Autodesk Inventor part; units mm, degrees
note: some values were not read from the file. Chosen so that the rebuilt part matches the saved one: direction of "Hole2".
(part 3 of 3)
  spline S120 degree 3 poles (-3.4442, 27.3191) (-3.5354, 27.4125) (-3.6453, 27.4727) (-3.7727, 27.4993) (-3.9002, 27.526) (-4.0253, 27.5146) (-4.1459, 27.4656) (-4.2665, 27.4166) (-4.3639, 27.3373) (-4.4367, 27.2293) (-4.5094, 27.1213) (-4.546, 27.0018) (-4.5461, 26.8709) knots 0 0 0 0 0.25 0.25 0.25 0.5 0.5 0.5 0.75 0.75 0.75 1 1 1 1
  spline S121 degree 3 poles (-5.388, 28.9585) (-5.3885, 28.9241) (-5.3861, 28.89) (-5.3809, 28.8564) knots 0 0 0 0 1 1 1 1
  line L115 (-4.5538, 28.7429) -> (-4.7042, 28.7429)
  spline S122 degree 3 poles (-5.3809, 28.8564) (-5.3777, 28.8422) (-5.3745, 28.8314) (-5.3727, 28.8257) (-5.3723, 28.8246) (-5.372, 28.8238) (-5.372, 28.8238) (-5.3718, 28.8234) (-5.3717, 28.8232) (-5.3716, 28.823) (-5.3715, 28.823) (-5.3715, 28.8229) (-5.3715, 28.8229) (-5.3715, 28.8229) (-5.3715, 28.8229) (-5.3715, 28.8229) (-5.3715, 28.8229) (-5.3715, 28.8229) (-5.3715, 28.8229) (-5.3715, 28.8229) (-5.3715, 28.823) (-5.3714, 28.823) (-5.3714, 28.823) (-5.3714, 28.8231) (-5.3714, 28.8232) (-5.3715, 28.8244) (-5.3721, 28.8277) (-5.3775, 28.8551) (-5.3859, 28.896) (-5.388, 28.9585) knots 0 0 0 0 0.216458 0.216458 0.250147 0.250147 0.25213 0.25213 0.266562 0.266562 0.270758 0.270758 0.271952 0.271952 0.272738 0.272738 0.27341 0.27341 0.274154 0.274154 0.275352 0.275352 0.277883 0.277883 0.289351 0.289351 0.40678 0.40678 1 1 1 1
  line L116 (-4.7883, 28.3589) -> (-4.4696, 28.3589)
  line L117 (-4.7883, 28.3589) -> (-4.4696, 28.3589)
  spline S123 degree 3 poles (-4.4696, 28.3589) (-4.4353, 28.359) (-4.4013, 28.3621) (-4.3679, 28.3678) knots 0 0 0 0 1 1 1 1
  spline S124 degree 3 poles (-4.3679, 28.3678) (-4.3538, 28.3714) (-4.343, 28.3747) (-4.3374, 28.3767) (-4.3363, 28.3771) (-4.3355, 28.3774) (-4.3355, 28.3774) (-4.3351, 28.3776) (-4.3349, 28.3777) (-4.3347, 28.3778) (-4.3347, 28.3779) (-4.3346, 28.3779) (-4.3346, 28.3779) (-4.3346, 28.3779) (-4.3346, 28.3779) (-4.3346, 28.3779) (-4.3346, 28.3779) (-4.3346, 28.3779) (-4.3346, 28.3779) (-4.3347, 28.3779) (-4.3347, 28.3779) (-4.3347, 28.378) (-4.3347, 28.378) (-4.3348, 28.378) (-4.3349, 28.378) (-4.3361, 28.3779) (-4.3393, 28.3772) (-4.3666, 28.3713) (-4.4073, 28.3622) (-4.4696, 28.3589) knots 0 0 0 0 0.216458 0.216458 0.250147 0.250147 0.25213 0.25213 0.266562 0.266562 0.270758 0.270758 0.271952 0.271952 0.272738 0.272738 0.27341 0.27341 0.274155 0.274155 0.275353 0.275353 0.277883 0.277883 0.289351 0.289351 0.40678 0.40678 1 1 1 1
  spline S125 degree 3 poles (-4.3679, 28.3678) (-4.3232, 28.3756) (-4.2796, 28.3882) (-4.2022, 28.4204) (-4.168, 28.4387) (-4.1034, 28.482) (-4.0717, 28.5083) (-4.0175, 28.5623) (-3.9933, 28.5919) (-3.9503, 28.6563) (-3.931, 28.6927) (-3.8857, 28.8003) (-3.8704, 28.8769) (-3.87, 28.9585) knots 0.106772 0.106772 0.106772 0.106772 0.25 0.25 0.375 0.375 0.5 0.5 0.625 0.625 0.75 0.75 1 1 1 1
  spline S126 degree 3 poles (-4.4696, 28.3589) (-4.3893, 28.3592) (-4.3104, 28.3755) (-4.2022, 28.4204) (-4.168, 28.4387) (-4.1034, 28.482) (-4.0717, 28.5083) (-4.0175, 28.5623) (-3.9933, 28.5919) (-3.9503, 28.6563) (-3.931, 28.6927) (-3.8857, 28.8003) (-3.8704, 28.8769) (-3.87, 28.9585) knots 0 0 0 0 0.25 0.25 0.375 0.375 0.5 0.5 0.625 0.625 0.75 0.75 1 1 1 1
  spline S127 degree 3 poles (-5.3809, 28.8564) (-5.3731, 28.8116) (-5.3603, 28.7681) (-5.328, 28.6905) (-5.3096, 28.6563) (-5.2661, 28.5918) (-5.2397, 28.5601) (-5.1855, 28.5059) (-5.1558, 28.4816) (-5.0912, 28.4388) (-5.0547, 28.4195) (-4.9469, 28.3743) (-4.8701, 28.3591) (-4.7883, 28.3589) knots 0.106772 0.106772 0.106772 0.106772 0.25 0.25 0.375 0.375 0.5 0.5 0.625 0.625 0.75 0.75 1 1 1 1
  spline S128 degree 3 poles (-3.4442, 27.3191) (-3.5354, 27.4125) (-3.6453, 27.4727) (-3.7727, 27.4993) (-3.9002, 27.526) (-4.0253, 27.5146) (-4.1459, 27.4656) (-4.2665, 27.4166) (-4.3639, 27.3373) (-4.4367, 27.2293) (-4.5094, 27.1213) (-4.546, 27.0018) (-4.5461, 26.8709) knots 0 0 0 0 0.25 0.25 0.25 0.5 0.5 0.5 0.75 0.75 0.75 1 1 1 1
  spline S129 degree 3 poles (-5.388, 28.9585) (-5.3876, 28.8781) (-5.3714, 28.7993) (-5.3265, 28.691) (-5.3082, 28.6569) (-5.2649, 28.5923) (-5.2385, 28.5606) (-5.1846, 28.5064) (-5.155, 28.4821) (-5.0906, 28.4392) (-5.0541, 28.4199) (-4.9466, 28.3745) (-4.8699, 28.3592) (-4.7883, 28.3589) knots 0 0 0 0 0.25 0.25 0.375 0.375 0.5 0.5 0.625 0.625 0.75 0.75 1 1 1 1
  spline S130 degree 3 poles (-1.886, 26.4062) (-2.182, 26.4856) (-2.4626, 26.6029) (-2.7267, 26.7575) (-2.9908, 26.9122) (-3.23, 27.0994) (-3.4442, 27.3191) knots 0 0 0 0 0.5 0.5 0.5 1 1 1 1
  spline S131 degree 3 poles (-1.886, 26.4062) (-2.182, 26.4856) (-2.4626, 26.6029) (-2.7267, 26.7575) (-2.9908, 26.9122) (-3.23, 27.0994) (-3.4442, 27.3191) knots 0 0 0 0 0.5 0.5 0.5 1 1 1 1
  arc A62 (-3.254, 29.698) -> (1.246, 29.698) centre (-1.004, 29.698) ccw
  arc A63 (-3.254, 29.698) -> (1.246, 29.698) centre (-1.004, 29.698) ccw
  spline S132 degree 3 poles (2.4039, 29.698) (2.4039, 29.5157) (2.3896, 29.3357) (2.3611, 29.158) (2.3468, 29.0691) (2.329, 28.9808) (2.3076, 28.8931) (2.2969, 28.8492) (2.2854, 28.8055) (2.2729, 28.7619) (2.2666, 28.7401) (2.2602, 28.7184) (2.2535, 28.6967) (2.2468, 28.675) (2.2403, 28.6545) (2.2328, 28.6316) (2.1123, 28.2657) (1.9342, 27.929) (1.6997, 27.6234) (1.5825, 27.4705) (1.4542, 27.3295) (1.3149, 27.2001) (1.2452, 27.1355) (1.1728, 27.0738) (1.0976, 27.015) (1.06, 26.9856) (1.0217, 26.957) (0.9828, 26.929) (0.9633, 26.9151) (0.9436, 26.9013) (0.9238, 26.8877) (0.904, 26.8741) (0.8828, 26.86) (0.8638, 26.8475) (0.5591, 26.6478) (0.2306, 26.5007) (-0.1219, 26.4062) knots 0 0 0 0 0.125 0.125 0.125 0.1875 0.1875 0.1875 0.21875 0.21875 0.21875 0.234375 0.234375 0.234375 0.25 0.25 0.25 0.5 0.5 0.5 0.625 0.625 0.625 0.6875 0.6875 0.6875 0.71875 0.71875 0.71875 0.734375 0.734375 0.734375 0.75 0.75 0.75 1 1 1 1
  line L118 (2.4039, 30.098) -> (2.4039, 29.698)
  arc A64 (-0.0226, 26.0353) -> (-0.3621, 25.5928) centre (0.096, 25.5928) ccw
  line L119 (4.5381, 25.998) -> (4.5381, 30.098)
  line L120 (4.5381, 25.998) -> (4.5381, 30.098)
  line L121 (4.1541, 25.998) -> (4.1541, 30.098)
  line L122 (2.7879, 29.698) -> (2.7879, 30.098)
  line L123 (2.4039, 30.098) -> (2.4039, 29.698)
  spline S133 degree 3 poles (2.4039, 29.698) (2.4039, 29.5157) (2.3896, 29.3357) (2.3611, 29.158) (2.3468, 29.0691) (2.329, 28.9808) (2.3076, 28.8931) (2.2969, 28.8492) (2.2854, 28.8055) (2.2729, 28.7619) (2.2666, 28.7401) (2.2602, 28.7184) (2.2535, 28.6967) (2.2468, 28.675) (2.2403, 28.6545) (2.2328, 28.6316) (2.1123, 28.2657) (1.9342, 27.929) (1.6997, 27.6234) (1.5825, 27.4705) (1.4542, 27.3295) (1.3149, 27.2001) (1.2452, 27.1355) (1.1728, 27.0738) (1.0976, 27.015) (1.06, 26.9856) (1.0217, 26.957) (0.9828, 26.929) (0.9633, 26.9151) (0.9436, 26.9013) (0.9238, 26.8877) (0.904, 26.8741) (0.8828, 26.86) (0.8638, 26.8475) (0.5591, 26.6478) (0.2306, 26.5007) (-0.1219, 26.4062) knots 0 0 0 0 0.125 0.125 0.125 0.1875 0.1875 0.1875 0.21875 0.21875 0.21875 0.234375 0.234375 0.234375 0.25 0.25 0.25 0.5 0.5 0.5 0.625 0.625 0.625 0.6875 0.6875 0.6875 0.71875 0.71875 0.71875 0.734375 0.734375 0.734375 0.75 0.75 0.75 1 1 1 1
  arc A65 (-0.0226, 26.0353) -> (2.7879, 29.698) centre (-1.004, 29.698) ccw
  line L124 (1.246, 29.698) -> (1.246, 32.698)
  line L125 (1.246, 32.698) -> (1.246, 29.698)
  spline S134 degree 3 poles (4.5381, 30.098) (4.5381, 30.1515) (4.533, 30.2041) (4.5232, 30.2558) (4.5183, 30.2816) (4.5121, 30.3072) (4.5048, 30.3326) (4.4974, 30.3579) (4.4896, 30.381) (4.479, 30.4079) (4.4363, 30.5157) (4.3734, 30.6114) (4.2914, 30.6934) (4.2505, 30.7344) (4.2061, 30.7704) (4.1585, 30.8017) (4.1348, 30.8173) (4.1102, 30.8317) (4.0848, 30.845) (4.072, 30.8516) (4.0591, 30.8579) (4.046, 30.8639) (4.0329, 30.8699) (4.0184, 30.876) (4.006, 30.8809) (3.9067, 30.9202) (3.8034, 30.94) (3.696, 30.9401) knots 0 0 0 0 0.125 0.125 0.125 0.1875 0.1875 0.1875 0.25 0.25 0.25 0.5 0.5 0.5 0.625 0.625 0.625 0.6875 0.6875 0.6875 0.71875 0.71875 0.71875 0.75 0.75 0.75 1 1 1 1
  spline S135 degree 3 poles (3.696, 31.4559) (3.7495, 31.4559) (3.8021, 31.461) (3.8538, 31.4708) (3.8796, 31.4757) (3.9052, 31.4819) (3.9306, 31.4892) (3.956, 31.4966) (3.979, 31.5044) (4.006, 31.515) (4.1138, 31.5577) (4.2094, 31.6206) (4.2914, 31.7026) (4.3324, 31.7435) (4.3684, 31.7879) (4.3997, 31.8354) (4.4153, 31.8592) (4.4298, 31.8838) (4.443, 31.9092) (4.4496, 31.9219) (4.4559, 31.9349) (4.4619, 31.948) (4.4679, 31.9611) (4.4741, 31.9756) (4.479, 31.988) (4.5183, 32.0873) (4.538, 32.1906) (4.5381, 32.298) knots 0 0 0 0 0.125 0.125 0.125 0.1875 0.1875 0.1875 0.25 0.25 0.25 0.5 0.5 0.5 0.625 0.625 0.625 0.6875 0.6875 0.6875 0.71875 0.71875 0.71875 0.75 0.75 0.75 1 1 1 1
  line L126 (3.696, 30.9401) -> (3.246, 30.9401)
  line L127 (3.246, 31.4559) -> (3.696, 31.4559)
  spline S136 degree 3 poles (3.246, 30.9401) (3.1925, 30.94) (3.1399, 30.9351) (3.0882, 30.9252) (3.0624, 30.9203) (3.0368, 30.9142) (3.0114, 30.9068) (2.9861, 30.8994) (2.963, 30.8916) (2.936, 30.8809) (2.8282, 30.8383) (2.7326, 30.7753) (2.6506, 30.6934) (2.6096, 30.6525) (2.5734, 30.6082) (2.5422, 30.5606) (2.5266, 30.5368) (2.5121, 30.5122) (2.499, 30.4868) (2.4924, 30.474) (2.4861, 30.4611) (2.4801, 30.448) (2.4741, 30.4348) (2.468, 30.4203) (2.4631, 30.4079) (2.4237, 30.3087) (2.404, 30.2054) (2.4039, 30.098) knots 0 0 0 0 0.125 0.125 0.125 0.1875 0.1875 0.1875 0.25 0.25 0.25 0.5 0.5 0.5 0.625 0.625 0.625 0.6875 0.6875 0.6875 0.71875 0.71875 0.71875 0.75 0.75 0.75 1 1 1 1
  line L128 (3.696, 30.5561) -> (3.246, 30.5561)
  arc A66 (4.1541, 30.098) -> (3.696, 30.5561) centre (3.696, 30.098) ccw
  arc A67 (3.246, 30.5561) -> (2.7879, 30.098) centre (3.246, 30.098) ccw
  line L129 (3.696, 30.9401) -> (3.246, 30.9401)
  spline S137 degree 3 poles (4.5381, 30.098) (4.5381, 30.1515) (4.533, 30.2041) (4.5232, 30.2558) (4.5183, 30.2816) (4.5121, 30.3072) (4.5048, 30.3326) (4.4974, 30.3579) (4.4896, 30.381) (4.479, 30.4079) (4.4363, 30.5157) (4.3734, 30.6114) (4.2914, 30.6934) (4.2505, 30.7344) (4.2061, 30.7704) (4.1585, 30.8017) (4.1348, 30.8173) (4.1102, 30.8317) (4.0848, 30.845) (4.072, 30.8516) (4.0591, 30.8579) (4.046, 30.8639) (4.0329, 30.8699) (4.0184, 30.876) (4.006, 30.8809) (3.9067, 30.9202) (3.8034, 30.94) (3.696, 30.9401) knots 0 0 0 0 0.125 0.125 0.125 0.1875 0.1875 0.1875 0.25 0.25 0.25 0.5 0.5 0.5 0.625 0.625 0.625 0.6875 0.6875 0.6875 0.71875 0.71875 0.71875 0.75 0.75 0.75 1 1 1 1
  line L130 (3.246, 31.4559) -> (3.696, 31.4559)
  line L131 (3.246, 31.8399) -> (3.696, 31.8399)
  spline S138 degree 3 poles (3.696, 31.4559) (3.7495, 31.4559) (3.8021, 31.461) (3.8538, 31.4708) (3.8796, 31.4757) (3.9052, 31.4819) (3.9306, 31.4892) (3.956, 31.4966) (3.979, 31.5044) (4.006, 31.515) (4.1138, 31.5577) (4.2094, 31.6206) (4.2914, 31.7026) (4.3324, 31.7435) (4.3684, 31.7879) (4.3997, 31.8354) (4.4153, 31.8592) (4.4298, 31.8838) (4.443, 31.9092) (4.4496, 31.9219) (4.4559, 31.9349) (4.4619, 31.948) (4.4679, 31.9611) (4.4741, 31.9756) (4.479, 31.988) (4.5183, 32.0873) (4.538, 32.1906) (4.5381, 32.298) knots 0 0 0 0 0.125 0.125 0.125 0.1875 0.1875 0.1875 0.25 0.25 0.25 0.5 0.5 0.5 0.625 0.625 0.625 0.6875 0.6875 0.6875 0.71875 0.71875 0.71875 0.75 0.75 0.75 1 1 1 1
  arc A68 (3.696, 31.8399) -> (4.1541, 32.298) centre (3.696, 32.298) ccw
  arc A69 (2.7879, 32.298) -> (3.246, 31.8399) centre (3.246, 32.298) ccw
  spline S139 degree 3 poles (2.4039, 32.298) (2.404, 32.2444) (2.4089, 32.1918) (2.4188, 32.1402) (2.4237, 32.1144) (2.4298, 32.0888) (2.4372, 32.0634) (2.4446, 32.038) (2.4524, 32.015) (2.4631, 31.988) (2.5057, 31.8802) (2.5687, 31.7846) (2.6506, 31.7025) (2.6915, 31.6615) (2.7358, 31.6254) (2.7834, 31.5942) (2.8072, 31.5785) (2.8318, 31.5641) (2.8572, 31.5509) (2.8699, 31.5443) (2.8829, 31.5381) (2.896, 31.5321) (2.9092, 31.5261) (2.9236, 31.5199) (2.936, 31.515) (3.0353, 31.4757) (3.1386, 31.456) (3.246, 31.4559) knots 0 0 0 0 0.125 0.125 0.125 0.1875 0.1875 0.1875 0.25 0.25 0.25 0.5 0.5 0.5 0.625 0.625 0.625 0.6875 0.6875 0.6875 0.71875 0.71875 0.71875 0.75 0.75 0.75 1 1 1 1
  spline S140 degree 3 poles (2.4039, 32.298) (2.404, 32.2444) (2.4089, 32.1918) (2.4188, 32.1402) (2.4237, 32.1144) (2.4298, 32.0888) (2.4372, 32.0634) (2.4446, 32.038) (2.4524, 32.015) (2.4631, 31.988) (2.5057, 31.8802) (2.5687, 31.7846) (2.6506, 31.7025) (2.6915, 31.6615) (2.7358, 31.6254) (2.7834, 31.5942) (2.8072, 31.5785) (2.8318, 31.5641) (2.8572, 31.5509) (2.8699, 31.5443) (2.8829, 31.5381) (2.896, 31.5321) (2.9092, 31.5261) (2.9236, 31.5199) (2.936, 31.515) (3.0353, 31.4757) (3.1386, 31.456) (3.246, 31.4559) knots 0 0 0 0 0.125 0.125 0.125 0.1875 0.1875 0.1875 0.25 0.25 0.25 0.5 0.5 0.5 0.625 0.625 0.625 0.6875 0.6875 0.6875 0.71875 0.71875 0.71875 0.75 0.75 0.75 1 1 1 1
  spline S141 degree 3 poles (3.246, 30.9401) (3.1925, 30.94) (3.1399, 30.9351) (3.0882, 30.9252) (3.0624, 30.9203) (3.0368, 30.9142) (3.0114, 30.9068) (2.9861, 30.8994) (2.963, 30.8916) (2.936, 30.8809) (2.8282, 30.8383) (2.7326, 30.7753) (2.6506, 30.6934) (2.6096, 30.6525) (2.5734, 30.6082) (2.5422, 30.5606) (2.5266, 30.5368) (2.5121, 30.5122) (2.499, 30.4868) (2.4924, 30.474) (2.4861, 30.4611) (2.4801, 30.448) (2.4741, 30.4348) (2.468, 30.4203) (2.4631, 30.4079) (2.4237, 30.3087) (2.404, 30.2054) (2.4039, 30.098) knots 0 0 0 0 0.125 0.125 0.125 0.1875 0.1875 0.1875 0.25 0.25 0.25 0.5 0.5 0.5 0.625 0.625 0.625 0.6875 0.6875 0.6875 0.71875 0.71875 0.71875 0.75 0.75 0.75 1 1 1 1
  ellipse E14 centre (-4.7038, 29.043) end of major axis (-4.4914, 29.2554) minor radius 0.3 (-5.004, 29.0427) -> (-4.7042, 28.7429) ccw
  ellipse E15 centre (-4.5542, 29.043) end of major axis (-4.7666, 29.2554) minor radius 0.3 (-4.5538, 28.7429) -> (-4.254, 29.0427) ccw
  line L132 (-5.388, 33.4375) -> (-5.388, 28.9585)
  line L133 (-5.388, 33.4375) -> (-5.388, 28.9585)
  line L134 (-5.004, 29.0427) -> (-5.004, 33.3533)
  line L135 (-4.254, 33.3533) -> (-4.254, 29.0427)
  line L136 (-3.87, 28.9585) -> (-3.87, 33.4375)
  line L137 (-3.87, 28.9585) -> (-3.87, 33.4375)
  line L138 (-3.254, 32.698) -> (-3.254, 29.698)
  line L139 (-3.254, 29.698) -> (-3.254, 32.698)
  spline S142 degree 3 poles (-3.87, 33.4375) (-3.8702, 33.4718) (-3.8732, 33.5058) (-3.879, 33.5392) knots 0 0 0 0 1 1 1 1
  spline S143 degree 3 poles (-3.879, 33.5392) (-3.8825, 33.5533) (-3.8858, 33.564) (-3.8878, 33.5697) (-3.8882, 33.5708) (-3.8885, 33.5716) (-3.8885, 33.5716) (-3.8887, 33.572) (-3.8888, 33.5722) (-3.889, 33.5724) (-3.889, 33.5724) (-3.889, 33.5725) (-3.889, 33.5725) (-3.889, 33.5725) (-3.889, 33.5725) (-3.889, 33.5725) (-3.8891, 33.5725) (-3.8891, 33.5725) (-3.8891, 33.5724) (-3.8891, 33.5724) (-3.8891, 33.5724) (-3.8891, 33.5724) (-3.8891, 33.5724) (-3.8891, 33.5723) (-3.8891, 33.5722) (-3.889, 33.571) (-3.8883, 33.5678) (-3.8824, 33.5405) (-3.8733, 33.4998) (-3.87, 33.4375) knots 0 0 0 0 0.216458 0.216458 0.250147 0.250147 0.25213 0.25213 0.266562 0.266562 0.270758 0.270758 0.271952 0.271952 0.272738 0.272738 0.27341 0.27341 0.274154 0.274154 0.275352 0.275352 0.277883 0.277883 0.289351 0.289351 0.40678 0.40678 1 1 1 1
  ellipse E16 centre (-4.7038, 33.3529) end of major axis (-4.9162, 33.5653) minor radius 0.3 (-4.7042, 33.6531) -> (-5.004, 33.3533) ccw
  ellipse E17 centre (-4.5542, 33.3529) end of major axis (-4.3418, 33.5653) minor radius 0.3 (-4.254, 33.3533) -> (-4.5538, 33.6531) ccw
  line L140 (-4.7042, 33.6531) -> (-4.5538, 33.6531)
  spline S144 degree 3 poles (-3.879, 33.5392) (-3.8867, 33.5839) (-3.8994, 33.6275) (-3.9315, 33.7049) (-3.9498, 33.7391) (-3.9931, 33.8036) (-4.0194, 33.8354) (-4.0734, 33.8896) (-4.103, 33.9138) (-4.1674, 33.9567) (-4.2038, 33.9761) (-4.3114, 34.0214) (-4.388, 34.0367) (-4.4696, 34.0371) knots 0.106772 0.106772 0.106772 0.106772 0.25 0.25 0.375 0.375 0.5 0.5 0.625 0.625 0.75 0.75 1 1 1 1
  spline S145 degree 3 poles (-3.87, 33.4375) (-3.8704, 33.5178) (-3.8866, 33.5966) (-3.9315, 33.7049) (-3.9498, 33.7391) (-3.9931, 33.8036) (-4.0194, 33.8354) (-4.0734, 33.8896) (-4.103, 33.9138) (-4.1674, 33.9567) (-4.2038, 33.9761) (-4.3114, 34.0214) (-4.388, 34.0367) (-4.4696, 34.0371) knots 0 0 0 0 0.25 0.25 0.375 0.375 0.5 0.5 0.625 0.625 0.75 0.75 1 1 1 1
  spline S146 degree 3 poles (-4.8901, 34.0281) (-4.9042, 34.0246) (-4.9149, 34.0213) (-4.9206, 34.0193) (-4.9217, 34.0189) (-4.9224, 34.0186) (-4.9225, 34.0185) (-4.9229, 34.0184) (-4.9231, 34.0183) (-4.9233, 34.0181) (-4.9233, 34.0181) (-4.9233, 34.0181) (-4.9233, 34.0181) (-4.9233, 34.0181) (-4.9233, 34.0181) (-4.9233, 34.018) (-4.9233, 34.018) (-4.9233, 34.018) (-4.9233, 34.018) (-4.9233, 34.018) (-4.9233, 34.018) (-4.9233, 34.018) (-4.9233, 34.018) (-4.9232, 34.018) (-4.923, 34.018) (-4.9218, 34.0181) (-4.9186, 34.0188) (-4.8914, 34.0247) (-4.8507, 34.0338) (-4.7883, 34.0371) knots 0 0 0 0 0.216458 0.216458 0.250147 0.250147 0.25213 0.25213 0.266562 0.266562 0.270758 0.270758 0.271952 0.271952 0.272738 0.272738 0.27341 0.27341 0.274154 0.274154 0.275352 0.275352 0.277883 0.277883 0.289351 0.289351 0.40678 0.40678 1 1 1 1
  spline S147 degree 3 poles (-4.8901, 34.0281) (-4.9348, 34.0204) (-4.9784, 34.0077) (-5.0558, 33.9756) (-5.09, 33.9573) (-5.1545, 33.914) (-5.1862, 33.8877) (-5.2404, 33.8337) (-5.2647, 33.8041) (-5.3076, 33.7397) (-5.3269, 33.7032) (-5.3723, 33.5957) (-5.3876, 33.519) (-5.388, 33.4375) knots 0.106772 0.106772 0.106772 0.106772 0.25 0.25 0.375 0.375 0.5 0.5 0.625 0.625 0.75 0.75 1 1 1 1
  spline S148 degree 3 poles (-4.7883, 34.0371) (-4.8687, 34.0367) (-4.9475, 34.0205) (-5.0558, 33.9756) (-5.09, 33.9573) (-5.1545, 33.914) (-5.1862, 33.8877) (-5.2404, 33.8337) (-5.2647, 33.8041) (-5.3076, 33.7397) (-5.3269, 33.7032) (-5.3723, 33.5957) (-5.3876, 33.519) (-5.388, 33.4375) knots 0 0 0 0 0.25 0.25 0.375 0.375 0.5 0.5 0.625 0.625 0.75 0.75 1 1 1 1
  arc A70 (1.246, 32.698) -> (-3.254, 32.698) centre (-1.004, 32.698) ccw
  arc A71 (1.246, 32.698) -> (-3.254, 32.698) centre (-1.004, 32.698) ccw
  line L141 (-4.4696, 34.0371) -> (-4.7883, 34.0371)
  line L142 (-4.4696, 34.0371) -> (-4.7883, 34.0371)
  arc A72 (-4.0696, 35.6555) -> (-3.6357, 35.4279) centre (-3.8149, 35.6137) ccw
  spline S149 degree 3 poles (-4.4485, 35.7175) (-4.4707, 35.5811) (-4.4509, 35.4507) (-4.3894, 35.3271) (-4.328, 35.2036) (-4.2352, 35.1093) (-4.1131, 35.0451) (-3.991, 34.9809) (-3.8606, 34.9587) (-3.724, 34.9781) (-3.5874, 34.9975) (-3.4691, 35.0553) (-3.3692, 35.1515) knots 0 0 0 0 0.25 0.25 0.25 0.5 0.5 0.5 0.75 0.75 0.75 1 1 1 1
  spline S150 degree 3 poles (-4.4485, 35.7175) (-4.4707, 35.5811) (-4.4509, 35.4507) (-4.3894, 35.3271) (-4.328, 35.2036) (-4.2352, 35.1093) (-4.1131, 35.0451) (-3.991, 34.9809) (-3.8606, 34.9587) (-3.724, 34.9781) (-3.5874, 34.9975) (-3.4691, 35.0553) (-3.3692, 35.1515) knots 0 0 0 0 0.25 0.25 0.25 0.5 0.5 0.5 0.75 0.75 0.75 1 1 1 1
  spline S151 degree 3 poles (-4.7883, 34.0371) (-4.8227, 34.0369) (-4.8567, 34.0339) (-4.8901, 34.0281) knots 0 0 0 0 1 1 1 1
  spline S152 degree 3 poles (6.996, 35.6559) (7.0495, 35.6559) (7.1021, 35.6609) (7.1538, 35.6707) (7.1796, 35.6757) (7.2052, 35.6818) (7.2306, 35.6892) (7.256, 35.6966) (7.279, 35.7044) (7.306, 35.715) (7.4138, 35.7576) (7.5094, 35.8206) (7.5914, 35.9025) (7.6325, 35.9435) (7.6686, 35.9878) (7.6998, 36.0353) (7.7155, 36.0591) (7.7299, 36.0838) (7.7431, 36.1092) (7.7497, 36.1219) (7.7559, 36.1349) (7.7619, 36.148) (7.7679, 36.1611) (7.774, 36.1756) (7.779, 36.188) (7.8183, 36.2872) (7.838, 36.3906) (7.8381, 36.498) knots 0 0 0 0 0.125 0.125 0.125 0.1875 0.1875 0.1875 0.25 0.25 0.25 0.5 0.5 0.5 0.625 0.625 0.625 0.6875 0.6875 0.6875 0.71875 0.71875 0.71875 0.75 0.75 0.75 1 1 1 1
  arc A73 (9.8138, 37.1517) -> (9.8085, 36.998) centre (12.0442, 36.9978) ccw
  arc A74 (14.1781, 36.8443) -> (14.1835, 36.998) centre (11.9808, 36.9977) ccw
  arc A75 (14.1781, 36.8443) -> (14.1835, 36.998) centre (11.9808, 36.9977) ccw
  spline S153 degree 3 poles (9.8085, 36.998) (9.8086, 36.7263) (9.8575, 36.4639) (9.9551, 36.2108) (9.9673, 36.1791) (9.9818, 36.1439) (9.9966, 36.1105) (10.0114, 36.077) (10.0269, 36.0441) (10.0433, 36.0116) (10.0759, 35.9467) (10.1116, 35.8838) (10.1504, 35.8229) (10.228, 35.701) (10.3178, 35.5871) (10.4199, 35.4811) (10.624, 35.2692) (10.8627, 35.1037) (11.1327, 34.988) (11.1665, 34.9736) (11.2, 34.9602) (11.2317, 34.9484) (11.2634, 34.9365) (11.2952, 34.9254) (11.3271, 34.9151) (11.3911, 34.8945) (11.4556, 34.8769) (11.5208, 34.8624) (11.6511, 34.8334) (11.7838, 34.8165) (11.9189, 34.8118) (12.054, 34.8072) (12.1894, 34.8147) (12.3215, 34.8345) (12.4535, 34.8543) (12.5833, 34.8863) (12.7109, 34.9306) (12.8385, 34.9748) (12.9761, 35.0367) (13.1009, 35.1096) (13.2258, 35.1825) (13.3428, 35.2677) (13.4517, 35.3651) (13.5607, 35.4625) (13.661, 35.5715) (13.7478, 35.6873) (13.8346, 35.803) (13.9093, 35.9268) (13.9717, 36.0588) (13.9874, 36.0918) (14.0022, 36.1253) (14.0163, 36.1592) (14.0304, 36.1932) (14.0426, 36.2249) (14.0541, 36.2566) (14.077, 36.3201) (14.0969, 36.3842) (14.1137, 36.4489) (14.1474, 36.5783) (14.1689, 36.7101) (14.1781, 36.8443) knots 0 0 0 0 0.122106 0.122106 0.122106 0.137369 0.137369 0.137369 0.152633 0.152633 0.152633 0.183159 0.183159 0.183159 0.244212 0.244212 0.244212 0.366318 0.366318 0.366318 0.381581 0.381581 0.381581 0.396845 0.396845 0.396845 0.427371 0.427371 0.427371 0.488424 0.488424 0.488424 0.549477 0.549477 0.549477 0.61053 0.61053 0.61053 0.671583 0.671583 0.671583 0.732636 0.732636 0.732636 0.793689 0.793689 0.793689 0.854742 0.854742 0.854742 0.870005 0.870005 0.870005 0.885269 0.885269 0.885269 0.915795 0.915795 0.915795 0.976848 0.976848 0.976848 0.976848
  spline S154 degree 3 poles (9.8085, 36.998) (9.8086, 36.7263) (9.8575, 36.4639) (9.9551, 36.2108) (9.9673, 36.1791) (9.9818, 36.1439) (9.9966, 36.1105) (10.0114, 36.077) (10.0269, 36.0441) (10.0433, 36.0116) (10.0759, 35.9467) (10.1116, 35.8838) (10.1504, 35.8229) (10.228, 35.701) (10.3178, 35.5871) (10.4199, 35.4811) (10.624, 35.2692) (10.8627, 35.1037) (11.1327, 34.988) (11.1665, 34.9736) (11.2, 34.9602) (11.2317, 34.9484) (11.2634, 34.9365) (11.2952, 34.9254) (11.3271, 34.9151) (11.3911, 34.8945) (11.4556, 34.8769) (11.5208, 34.8624) (11.6511, 34.8334) (11.7838, 34.8165) (11.9189, 34.8118) (12.054, 34.8072) (12.1894, 34.8147) (12.3215, 34.8345) (12.4535, 34.8543) (12.5833, 34.8863) (12.7109, 34.9306) (12.8385, 34.9748) (12.9761, 35.0367) (13.1009, 35.1096) (13.2258, 35.1825) (13.3428, 35.2677) (13.4517, 35.3651) (13.5607, 35.4625) (13.661, 35.5715) (13.7478, 35.6873) (13.8346, 35.803) (13.9093, 35.9268) (13.9717, 36.0588) (13.9874, 36.0918) (14.0022, 36.1253) (14.0163, 36.1592) (14.0304, 36.1932) (14.0426, 36.2249) (14.0541, 36.2566) (14.077, 36.3201) (14.0969, 36.3842) (14.1137, 36.4489) (14.1474, 36.5783) (14.1689, 36.7101) (14.1781, 36.8443) knots 0 0 0 0 0.122106 0.122106 0.122106 0.137369 0.137369 0.137369 0.152633 0.152633 0.152633 0.183159 0.183159 0.183159 0.244212 0.244212 0.244212 0.366318 0.366318 0.366318 0.381581 0.381581 0.381581 0.396845 0.396845 0.396845 0.427371 0.427371 0.427371 0.488424 0.488424 0.488424 0.549477 0.549477 0.549477 0.61053 0.61053 0.61053 0.671583 0.671583 0.671583 0.732636 0.732636 0.732636 0.793689 0.793689 0.793689 0.854742 0.854742 0.854742 0.870005 0.870005 0.870005 0.885269 0.885269 0.885269 0.915795 0.915795 0.915795 0.976848 0.976848 0.976848 0.976848
  arc A76 (6.996, 36.0399) -> (7.4541, 36.498) centre (6.996, 36.498) ccw
  spline S155 degree 3 poles (6.996, 35.6559) (7.0495, 35.6559) (7.1021, 35.6609) (7.1538, 35.6707) (7.1796, 35.6757) (7.2052, 35.6818) (7.2306, 35.6892) (7.256, 35.6966) (7.279, 35.7044) (7.306, 35.715) (7.4138, 35.7576) (7.5094, 35.8206) (7.5914, 35.9025) (7.6325, 35.9435) (7.6686, 35.9878) (7.6998, 36.0353) (7.7155, 36.0591) (7.7299, 36.0838) (7.7431, 36.1092) (7.7497, 36.1219) (7.7559, 36.1349) (7.7619, 36.148) (7.7679, 36.1611) (7.774, 36.1756) (7.779, 36.188) (7.8183, 36.2872) (7.838, 36.3906) (7.8381, 36.498) knots 0 0 0 0 0.125 0.125 0.125 0.1875 0.1875 0.1875 0.25 0.25 0.25 0.5 0.5 0.5 0.625 0.625 0.625 0.6875 0.6875 0.6875 0.71875 0.71875 0.71875 0.75 0.75 0.75 1 1 1 1
  line L143 (5.196, 36.0399) -> (6.996, 36.0399)
  line L144 (5.196, 35.6559) -> (6.996, 35.6559)
  line L145 (5.196, 35.6559) -> (6.996, 35.6559)
  spline S156 degree 3 poles (14.1835, 36.998) (14.1834, 37.2697) (14.1346, 37.5321) (14.0369, 37.7852) (14.0247, 37.8168) (14.0102, 37.852) (13.9954, 37.8855) (13.9807, 37.9189) (13.9651, 37.9519) (13.9488, 37.9843) (13.9161, 38.0492) (13.8804, 38.1122) (13.8416, 38.1731) (13.7641, 38.295) (13.6742, 38.4089) (13.5722, 38.5148) (13.368, 38.7268) (13.1293, 38.8922) (12.8593, 39.0079) (12.8255, 39.0224) (12.792, 39.0358) (12.7603, 39.0476) (12.7287, 39.0595) (12.6968, 39.0705) (12.6649, 39.0808) (12.6009, 39.1015) (12.5364, 39.119) (12.4712, 39.1336) (12.341, 39.1626) (12.2082, 39.1795) (12.0731, 39.1841) (11.938, 39.1888) (11.8026, 39.1812) (11.6705, 39.1614) (11.5385, 39.1417) (11.4087, 39.1096) (11.2811, 39.0654) (11.1536, 39.0212) (11.016, 38.9593) (10.8911, 38.8864) (10.7662, 38.8135) (10.6493, 38.7283) (10.5403, 38.6309) (10.4313, 38.5334) (10.331, 38.4245) (10.2442, 38.3087) (10.1574, 38.193) (10.0828, 38.0691) (10.0203, 37.9372) (10.0047, 37.9042) (9.9898, 37.8707) (9.9757, 37.8367) (9.9616, 37.8027) (9.9494, 37.7711) (9.9379, 37.7393) (9.915, 37.6758) (9.8951, 37.6118) (9.8783, 37.5471) (9.8446, 37.4177) (9.8231, 37.2859) (9.8138, 37.1517) knots 0 0 0 0 0.122106 0.122106 0.122106 0.137369 0.137369 0.137369 0.152633 0.152633 0.152633 0.183159 0.183159 0.183159 0.244212 0.244212 0.244212 0.366318 0.366318 0.366318 0.381581 0.381581 0.381581 0.396845 0.396845 0.396845 0.427371 0.427371 0.427371 0.488424 0.488424 0.488424 0.549477 0.549477 0.549477 0.61053 0.61053 0.61053 0.671583 0.671583 0.671583 0.732636 0.732636 0.732636 0.793689 0.793689 0.793689 0.854742 0.854742 0.854742 0.870005 0.870005 0.870005 0.885269 0.885269 0.885269 0.915795 0.915795 0.915795 0.976848 0.976848 0.976848 0.976848
  arc A77 (9.8138, 37.1517) -> (9.8085, 36.998) centre (12.0442, 36.9978) ccw
  spline S157 degree 3 poles (14.1835, 36.998) (14.1834, 37.2697) (14.1346, 37.5321) (14.0369, 37.7852) (14.0247, 37.8168) (14.0102, 37.852) (13.9954, 37.8855) (13.9807, 37.9189) (13.9651, 37.9519) (13.9488, 37.9843) (13.9161, 38.0492) (13.8804, 38.1122) (13.8416, 38.1731) (13.7641, 38.295) (13.6742, 38.4089) (13.5722, 38.5148) (13.368, 38.7268) (13.1293, 38.8922) (12.8593, 39.0079) (12.8255, 39.0224) (12.792, 39.0358) (12.7603, 39.0476) (12.7287, 39.0595) (12.6968, 39.0705) (12.6649, 39.0808) (12.6009, 39.1015) (12.5364, 39.119) (12.4712, 39.1336) (12.341, 39.1626) (12.2082, 39.1795) (12.0731, 39.1841) (11.938, 39.1888) (11.8026, 39.1812) (11.6705, 39.1614) (11.5385, 39.1417) (11.4087, 39.1096) (11.2811, 39.0654) (11.1536, 39.0212) (11.016, 38.9593) (10.8911, 38.8864) (10.7662, 38.8135) (10.6493, 38.7283) (10.5403, 38.6309) (10.4313, 38.5334) (10.331, 38.4245) (10.2442, 38.3087) (10.1574, 38.193) (10.0828, 38.0691) (10.0203, 37.9372) (10.0047, 37.9042) (9.9898, 37.8707) (9.9757, 37.8367) (9.9616, 37.8027) (9.9494, 37.7711) (9.9379, 37.7393) (9.915, 37.6758) (9.8951, 37.6118) (9.8783, 37.5471) (9.8446, 37.4177) (9.8231, 37.2859) (9.8138, 37.1517) knots 0 0 0 0 0.122106 0.122106 0.122106 0.137369 0.137369 0.137369 0.152633 0.152633 0.152633 0.183159 0.183159 0.183159 0.244212 0.244212 0.244212 0.366318 0.366318 0.366318 0.381581 0.381581 0.381581 0.396845 0.396845 0.396845 0.427371 0.427371 0.427371 0.488424 0.488424 0.488424 0.549477 0.549477 0.549477 0.61053 0.61053 0.61053 0.671583 0.671583 0.671583 0.732636 0.732636 0.732636 0.793689 0.793689 0.793689 0.854742 0.854742 0.854742 0.870005 0.870005 0.870005 0.885269 0.885269 0.885269 0.915795 0.915795 0.915795 0.976848 0.976848 0.976848 0.976848
  arc A78 (-1.6459, 39.3577) -> (-2.0872, 39.5394) centre (-1.904, 39.3577) ccw
  spline S158 degree 3 poles (-1.2619, 39.3577) (-1.262, 39.4877) (-1.2984, 39.6071) (-1.3705, 39.7149) (-1.4426, 39.8227) (-1.5396, 39.9018) (-1.6595, 39.9513) (-1.7794, 40.0007) (-1.904, 40.0126) (-2.0311, 39.987) (-2.1583, 39.9613) (-2.2679, 39.9024) (-2.3598, 39.8099) knots 0 0 0 0 0.25 0.25 0.25 0.5 0.5 0.5 0.75 0.75 0.75 1 1 1 1
  arc A79 (-0.1022, 40.9517) -> (-0.3621, 40.5387) centre (0.096, 40.5387) ccw
  spline S159 degree 3 poles (-0.2683, 41.2979) (-0.4142, 41.2277) (-0.5305, 41.1239) (-0.6166, 40.9872) (-0.7028, 40.8504) (-0.746, 40.7009) (-0.7461, 40.5387) knots 0 0 0 0 0.5 0.5 0.5 1 1 1 1
  spline S160 degree 3 poles (-0.2683, 41.2979) (-0.4142, 41.2277) (-0.5305, 41.1239) (-0.6166, 40.9872) (-0.7028, 40.8504) (-0.746, 40.7009) (-0.7461, 40.5387) knots 0 0 0 0 0.5 0.5 0.5 1 1 1 1
  spline S161 degree 3 poles (-1.2619, 39.3577) (-1.262, 39.4877) (-1.2984, 39.6071) (-1.3705, 39.7149) (-1.4426, 39.8227) (-1.5396, 39.9018) (-1.6595, 39.9513) (-1.7794, 40.0007) (-1.904, 40.0126) (-2.0311, 39.987) (-2.1583, 39.9613) (-2.2679, 39.9024) (-2.3598, 39.8099) knots 0 0 0 0 0.25 0.25 0.25 0.5 0.5 0.5 0.75 0.75 0.75 1 1 1 1
  line L146 (7.8381, 36.498) -> (7.8381, 41.198)
  line L147 (7.8381, 36.498) -> (7.8381, 41.198)
  line L148 (7.4541, 41.198) -> (7.4541, 36.498)
  line L149 (2.9943, 41.6561) -> (6.996, 41.6561)
  line L150 (6.996, 42.0401) -> (2.9943, 42.0401)
  line L151 (6.996, 42.0401) -> (2.9943, 42.0401)
  arc A80 (7.4541, 41.198) -> (6.996, 41.6561) centre (6.996, 41.198) ccw
  spline S162 degree 3 poles (7.8381, 41.198) (7.8381, 41.2515) (7.833, 41.3041) (7.8232, 41.3558) (7.8183, 41.3816) (7.8121, 41.4072) (7.8048, 41.4326) (7.7974, 41.4579) (7.7896, 41.481) (7.779, 41.5079) (7.7363, 41.6157) (7.6734, 41.7114) (7.5914, 41.7934) (7.5505, 41.8344) (7.5061, 41.8704) (7.4585, 41.9017) (7.4348, 41.9173) (7.4102, 41.9317) (7.3848, 41.945) (7.372, 41.9516) (7.3591, 41.9579) (7.346, 41.9639) (7.3329, 41.9699) (7.3184, 41.976) (7.306, 41.9809) (7.2067, 42.0202) (7.1034, 42.04) (6.996, 42.0401) knots 0 0 0 0 0.125 0.125 0.125 0.1875 0.1875 0.1875 0.25 0.25 0.25 0.5 0.5 0.5 0.625 0.625 0.625 0.6875 0.6875 0.6875 0.71875 0.71875 0.71875 0.75 0.75 0.75 1 1 1 1
  spline S163 degree 3 poles (7.8381, 41.198) (7.8381, 41.2515) (7.833, 41.3041) (7.8232, 41.3558) (7.8183, 41.3816) (7.8121, 41.4072) (7.8048, 41.4326) (7.7974, 41.4579) (7.7896, 41.481) (7.779, 41.5079) (7.7363, 41.6157) (7.6734, 41.7114) (7.5914, 41.7934) (7.5505, 41.8344) (7.5061, 41.8704) (7.4585, 41.9017) (7.4348, 41.9173) (7.4102, 41.9317) (7.3848, 41.945) (7.372, 41.9516) (7.3591, 41.9579) (7.346, 41.9639) (7.3329, 41.9699) (7.3184, 41.976) (7.306, 41.9809) (7.2067, 42.0202) (7.1034, 42.04) (6.996, 42.0401) knots 0 0 0 0 0.125 0.125 0.125 0.1875 0.1875 0.1875 0.25 0.25 0.25 0.5 0.5 0.5 0.625 0.625 0.625 0.6875 0.6875 0.6875 0.71875 0.71875 0.71875 0.75 0.75 0.75 1 1 1 1
  arc A81 (2.9943, 41.6561) -> (-0.1022, 40.9517) centre (2.9943, 34.498) ccw
  spline S164 degree 3 poles (2.9943, 42.0401) (2.4297, 42.04) (1.8716, 41.9773) (1.3214, 41.8522) (0.7711, 41.727) (0.2412, 41.5423) (-0.2683, 41.2979) knots 0 0 0 0 0.5 0.5 0.5 1 1 1 1
  spline S165 degree 3 poles (2.9943, 42.0401) (2.4297, 42.04) (1.8716, 41.9773) (1.3214, 41.8522) (0.7711, 41.727) (0.2412, 41.5423) (-0.2683, 41.2979) knots 0 0 0 0 0.5 0.5 0.5 1 1 1 1
  line L152 (2.4039, 32.698) -> (2.4039, 32.298)
  arc A82 (2.7879, 32.698) -> (-0.0226, 36.3607) centre (-1.004, 32.698) ccw
  spline S166 degree 3 poles (-0.1219, 35.9898) (0.0541, 35.9426) (0.2243, 35.8822) (0.3886, 35.8086) (0.4707, 35.7719) (0.5514, 35.7318) (0.6306, 35.6884) (0.6702, 35.6667) (0.7094, 35.6442) (0.7483, 35.6209) (0.7677, 35.6093) (0.7871, 35.5974) (0.8063, 35.5853) (0.8256, 35.5732) (0.8436, 35.5617) (0.8638, 35.5485) (1.186, 35.3374) (1.4652, 35.0782) (1.6997, 34.7726) (1.817, 34.6198) (1.92, 34.4594) (2.0089, 34.2913) (2.0533, 34.2073) (2.0942, 34.1214) (2.1315, 34.0335) (2.1502, 33.9896) (2.1679, 33.9452) (2.1848, 33.9004) (2.1933, 33.8779) (2.2015, 33.8554) (2.2095, 33.8327) (2.2175, 33.81) (2.2257, 33.786) (2.2328, 33.7643) (2.3468, 33.4184) (2.4039, 33.0629) (2.4039, 32.698) knots 0 0 0 0 0.125 0.125 0.125 0.1875 0.1875 0.1875 0.21875 0.21875 0.21875 0.234375 0.234375 0.234375 0.25 0.25 0.25 0.5 0.5 0.5 0.625 0.625 0.625 0.6875 0.6875 0.6875 0.71875 0.71875 0.71875 0.734375 0.734375 0.734375 0.75 0.75 0.75 1 1 1 1
  spline S167 degree 3 poles (-0.1219, 35.9898) (0.0541, 35.9426) (0.2243, 35.8822) (0.3886, 35.8086) (0.4707, 35.7719) (0.5514, 35.7318) (0.6306, 35.6884) (0.6702, 35.6667) (0.7094, 35.6442) (0.7483, 35.6209) (0.7677, 35.6093) (0.7871, 35.5974) (0.8063, 35.5853) (0.8256, 35.5732) (0.8436, 35.5617) (0.8638, 35.5485) (1.186, 35.3374) (1.4652, 35.0782) (1.6997, 34.7726) (1.817, 34.6198) (1.92, 34.4594) (2.0089, 34.2913) (2.0533, 34.2073) (2.0942, 34.1214) (2.1315, 34.0335) (2.1502, 33.9896) (2.1679, 33.9452) (2.1848, 33.9004) (2.1933, 33.8779) (2.2015, 33.8554) (2.2095, 33.8327) (2.2175, 33.81) (2.2257, 33.786) (2.2328, 33.7643) (2.3468, 33.4184) (2.4039, 33.0629) (2.4039, 32.698) knots 0 0 0 0 0.125 0.125 0.125 0.1875 0.1875 0.1875 0.21875 0.21875 0.21875 0.234375 0.234375 0.234375 0.25 0.25 0.25 0.5 0.5 0.5 0.625 0.625 0.625 0.6875 0.6875 0.6875 0.71875 0.71875 0.71875 0.734375 0.734375 0.734375 0.75 0.75 0.75 1 1 1 1
  line L153 (2.4039, 32.698) -> (2.4039, 32.298)
  line L154 (4.1541, 32.298) -> (4.1541, 34.998)
  line L155 (4.5381, 32.298) -> (4.5381, 34.998)
  line L156 (4.5381, 32.298) -> (4.5381, 34.998)
  arc A83 (5.196, 36.0399) -> (4.1541, 34.998) centre (5.196, 34.998) ccw
  spline S168 degree 3 poles (4.5381, 34.998) (4.5381, 35.0398) (4.542, 35.0809) (4.5497, 35.1213) (4.5535, 35.1414) (4.5584, 35.1614) (4.5641, 35.1813) (4.5699, 35.2011) (4.576, 35.2191) (4.5843, 35.2402) (4.6175, 35.3243) (4.6668, 35.3992) (4.7308, 35.4632) (4.7628, 35.4952) (4.7973, 35.5234) (4.8345, 35.5478) (4.8531, 35.5601) (4.8723, 35.5713) (4.8922, 35.5816) (4.9121, 35.5919) (4.9345, 35.602) (4.9538, 35.6097) (5.0313, 35.6404) (5.112, 35.6559) (5.196, 35.6559) knots 0 0 0 0 0.125 0.125 0.125 0.1875 0.1875 0.1875 0.25 0.25 0.25 0.5 0.5 0.5 0.625 0.625 0.625 0.6875 0.6875 0.6875 0.75 0.75 0.75 1 1 1 1
  spline S169 degree 3 poles (4.5381, 34.998) (4.5381, 35.0398) (4.542, 35.0809) (4.5497, 35.1213) (4.5535, 35.1414) (4.5584, 35.1614) (4.5641, 35.1813) (4.5699, 35.2011) (4.576, 35.2191) (4.5843, 35.2402) (4.6175, 35.3243) (4.6668, 35.3992) (4.7308, 35.4632) (4.7628, 35.4952) (4.7973, 35.5234) (4.8345, 35.5478) (4.8531, 35.5601) (4.8723, 35.5713) (4.8922, 35.5816) (4.9121, 35.5919) (4.9345, 35.602) (4.9538, 35.6097) (5.0313, 35.6404) (5.112, 35.6559) (5.196, 35.6559) knots 0 0 0 0 0.125 0.125 0.125 0.1875 0.1875 0.1875 0.25 0.25 0.25 0.5 0.5 0.5 0.625 0.625 0.625 0.6875 0.6875 0.6875 0.75 0.75 0.75 1 1 1 1
  line L157 (2.7879, 32.298) -> (2.7879, 32.698)
  point P0 (0, 0)
  point P1 (6.996, 18.498)
  constraints: 316 end point, 168 point on circle, 84 centre point, 442 other
extrude "Extrusion25" cut sketch "Sketch22" against normal up to next contours L83 A55 L109 A3 | L54 A19 L52 A17 | L138 A70 L124 A62
extrude "Extrusion26" cut sketch "Sketch22" against normal blind 2.6924 contours L87 E13 L98 E12 L85 E3 L19 E0 | A0 A7 L21 A39 A40 A41 L4 A6 | L6 A1 L7 A2 L10 A10 L29 A9 L26 A11 L32 A16 L41 A13 A14 L25 A8 A5 | L45 E4 L49 E5 L44 E2 L14 E1 | A12 L59 A22 L69 A34 L67 A35 L70 A36 A38 L74 A37 A21 L40 A15 L33 | A28 A31 L62 A30 A33 A29 | L80 A79 A81 L149 A80 L148 A76 L143 A83 L154 A68 L131 A69 L157 A82 A42 | A46 A72 A47 A78 L77 A43 | A64 A65 L122 A67 L128 A66 L121 A60 L112 A59 L103 A54 L106 A53 L111 A57 A58 L89 | L94 A49 A52 A51 L95 A61 A50 A48 | L115 E14 L134 E16 L140 E17 L135 E15
fillet "Fillet13" radius 0.3048 132 edges at (7.4541, 38.848, 0) (7.3199, 36.1741, 0) (6.096, 36.0399, 0) (4.4593, 35.7347, 0) (4.1541, 33.648, 0) (4.0199, 31.9741, 0) (3.471, 31.8399, 0) (2.9221, 31.9741, 0) (2.7879, 32.498, 0) (2.0043, 35.0063, 0) (-0.2674, 36.5243, 0) (-0.3621, 38.6709, 0) (-0.2917, 40.7827, 0) (1.4065, 41.4778, 0) (4.9952, 41.6561, 0) (7.3199, 41.5219, 0) (4.4593, 25.2612, 0) (6.096, 24.9561, 0) (7.3199, 24.8219, 0) (7.4541, 22.048, 0) (7.3199, 19.2741, 0) (5.121, 19.1399, 0) (2.9221, 19.2741, 0) (2.7879, 19.798, 0) (2.0043, 22.3063, 0) (-0.2674, 23.8243, 0) (-0.3621, 24.848, 0) (-0.2674, 25.8717, 0) (2.0043, 27.3896, 0) (2.7879, 29.898, 0) (2.9221, 30.4219, 0) (3.471, 30.5561, 0) (4.0199, 30.4219, 0) (4.1541, 28.048, 0) (7.4541, 14.948, 0) (7.3199, 12.1741, 0) (6.096, 12.0399, 0) (4.4593, 11.7347, 0) (4.1541, 8.948, 0) (4.0199, 6.5741, 0) (3.471, 6.4399, 0) (2.9221, 6.5741, 0) (2.7879, 7.098, 0) (2.0043, 9.6063, 0) (-0.2674, 11.1243, 0) (-0.3621, 12.148, 0) (-0.2674, 13.1717, 0) (2.0043, 14.6896, 0) (2.7879, 17.198, 0) (2.9221, 17.7219, 0) (5.121, 17.8561, 0) (7.3199, 17.7219, 0) (7.4541, -1.852, 0) (7.3199, -4.5259, 0) (4.9952, -4.6601, 0) (1.4065, -4.4818, 0) (-0.2917, -3.7867, 0) (-0.3621, -1.6749, 0) (-0.2674, 0.4717, 0) (2.0043, 1.9896, 0) (2.7879, 4.498, 0) (2.9221, 5.0219, 0) (3.471, 5.1561, 0) (4.0199, 5.0219, 0) (4.1541, 3.348, 0) (4.4593, 1.2612, 0) (6.096, 0.9561, 0) (7.3199, 0.8219, 0) (-1.6459, -1.0844, 0) (-1.8057, -2.6003, 0) (-3.3813, -0.7561, 0) (-3.9347, 1.6108, 0) (-2.8698, 0.9969, 0) (-1.7406, 0.4717, 0) (1.246, 5.798, 0) (-1.004, 2.048, 0) (-3.254, 5.798, 0) (-1.004, 9.548, 0) (-4.254, 5.798, 0) (-4.3418, 3.4307, 0) (-4.629, 3.3429, 0) (-4.9162, 3.4307, 0) (-5.004, 5.798, 0) (-4.9162, 8.1653, 0) (-4.629, 8.2531, 0) (-4.3418, 8.1653, 0) (-4.254, 18.498, 0) (-4.3418, 16.1307, 0) (-4.629, 16.0429, 0) (-4.9162, 16.1307, 0) (-5.004, 18.498, 0) (-4.9162, 20.8653, 0) (-4.629, 20.9531, 0) (-4.3418, 20.8653, 0) (-1.004, 14.748, 0) (-3.254, 18.498, 0) (-1.004, 22.248, 0) (1.246, 18.498, 0) (-1.6459, 12.148, 0) (-1.7406, 11.1243, 0) (-2.9208, 10.5697, 0) (-4.0012, 9.886, 0) (-4.1621, 12.148, 0) (-4.0012, 14.41, 0) (-2.9208, 13.7262, 0) (-1.7406, 13.1717, 0) (-1.6459, 24.848, 0) (-1.7406, 23.8243, 0) (-2.9208, 23.2697, 0) (-4.0012, 22.586, 0) (-4.1621, 24.848, 0) (-4.0012, 27.11, 0) (-2.9208, 26.4262, 0) (-1.7406, 25.8717, 0) (1.246, 31.198, 0) (-1.004, 27.448, 0) (-3.254, 31.198, 0) (-1.004, 34.948, 0) (-4.254, 31.198, 0) (-4.3418, 28.8307, 0) (-4.629, 28.7429, 0) (-4.9162, 28.8307, 0) (-5.004, 31.198, 0) (-4.9162, 33.5653, 0) (-4.629, 33.6531, 0) (-4.3418, 33.5653, 0) (-2.8698, 35.9991, 0) (-3.9347, 35.3852, 0) (-3.3813, 37.7521, 0) (-1.8057, 39.5963, 0) (-1.6459, 38.0804, 0) (-1.7406, 36.5243, 0)
fillet "Fillet14" radius 0.508 12 edges at (-1.004, 2.048, -4.4958) (1.246, 5.798, -4.4958) (-1.004, 9.548, -4.4958) (-3.254, 5.798, -4.4958) (-1.004, 14.748, -4.4958) (1.246, 18.498, -4.4958) (-1.004, 22.248, -4.4958) (-3.254, 18.498, -4.4958) (1.246, 31.198, -4.4958) (-1.004, 34.948, -4.4958) (-3.254, 31.198, -4.4958) (-1.004, 27.448, -4.4958)
fillet "Fillet15" radius 0.3048 5 edges at (-3.2269, -3.7115, -4.4958) (5.0969, -6.3428, -4.4958) (-5.8582, 18.5002, -4.4958) (-3.2269, 40.7119, -4.4958) (5.0969, 43.3432, -4.4958)
fillet "Fillet16" radius 0.3048 3 edges at (7.1531, -5.6646, -9.4996) (7.1531, 18.5071, -9.4996) (7.1531, 42.6758, -9.4996)
sketch "Sketch23" plane through (0, 0, 0) normal (0, 0, 1) x (1, 0, 0)
  circle A0 centre (55.4754, -0.0062) radius 1.0541
  circle A1 centre (55.4754, 36.9938) radius 1.0541
  circle A2 centre (55.4754, -0.0062) radius 1.8923
  circle A3 centre (55.4754, 36.9938) radius 1.8923
  point P0 (0, 0)
  dimension "d114" = 3.7846
  constraints: 2 centre point, 2 coincident, 1 equal radius
  measures "d114" diameter of A2
extrude "Extrusion27" cut sketch "Sketch23" against normal blind 2.794
fillet "Fillet17" radius 0.508 2 edges at (53.5831, -0.0062, 0) (53.5831, 36.9938, 0)
ref_plane "Work Plane4" through (16.9845, -4.5019, -3.81) normal (-1, 0, 0) x (0, -1, 0)
equation "\"d14\" = d12"
equation "\"d15\" = d12"
equation "\"d19\" = d16"
equation "\"d71\" = d69"
equation "\"d12\" = 0.6096"
body "Solid1"
